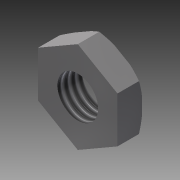
# Autodesk Inventor part: Nat(M4)
Saved by Autodesk Inventor 2013 (Build 170138000, 138)
## iProperties
Created: 2013-02-09
Material: ステンレス鋼
Document SubType Name: Modeling
Designer: andou
Density: 8.08 g/cm^3
Mass: 0.774277 g
Surface Area: 1.7348 cm^2
Volume: 0.0958263 cm^3
Author: andou
Title: Nat(M4)
Autodesk Inventor part; units mm, degrees
ref_plane "YZ Plane" through (0, 0, 0) normal (1, 0, 0) x (0, 1, 0)
ref_plane "XZ Plane" through (0, 0, 0) normal (0, 1, 0) x (-1, 0, 0)
ref_plane "XY Plane" through (0, 0, 0) normal (0, 0, 1) x (1, 0, 0)
sketch "スケッチ1" plane through (0, 0, 0) normal (0, 0, 1) x (1, 0, 0)
  line L0 (2, 1.2) -> (4, 1.2)
  line L1 (4.5, 0.9113) -> (4.5, -1.2)
  line L2 (4.5, -1.2) -> (2, -1.2)
  line L3 (2, -1.2) -> (2, 1.2)
  line L4 (0, 1.2) -> (0, -1.2)
  line L5 (4, 1.2) -> (4.5, 0.9113)
  point P0 (0, 0)
  dimension "d0" = 1.2
  dimension "d1" = 2.4
  dimension "d2" = 2
  dimension "d3" = 4.5
  dimension "d4" = 2
  dimension "d5" = 30
  constraints: 12 end point, 3 parallel, 1 horizontal, 1 perpendicular
  measures "d0" distance from line of point (0, 0) L0
  measures "d1" distance between parallel lines of L2 L0
  measures "d2" distance from line of point (0, 0) L3
  measures "d3" distance from line of point (0, 0) L1
  measures "d4" distance of L0.start L0.end
  measures "d5" angle of L0 L5
revolve "回転1" add sketch "スケッチ1" angle 360 about axis through (0, 1.2, 0) along (0, -1, 0)
sketch "スケッチ2" plane through (0, 1.2, 0) normal (0, 1, 0) x (1, 0, 0)
  circle A0 centre (0, 0) radius 2 projected
  line L0 (0, 4.5) -> (3.8971, 2.25)
  line L1 (3.8971, 2.25) -> (3.8971, -2.25)
  line L2 (3.8971, -2.25) -> (0, -4.5)
  line L3 (0, -4.5) -> (-3.8971, -2.25)
  line L4 (-3.8971, -2.25) -> (-3.8971, 2.25)
  line L5 (-3.8971, 2.25) -> (0, 4.5)
  dimension "d7" = 4.5
  constraints: 12 end point, 1 coincident, 13 other
  measures "d7" distance of point (0, 0) L0.start
extrude "押し出し1" cut sketch "スケッチ2" against normal blind 2.4 keep common part
thread "ねじ2" size "M4x0.7" class "6H" standard "ANSI Metric M Profile" full length
